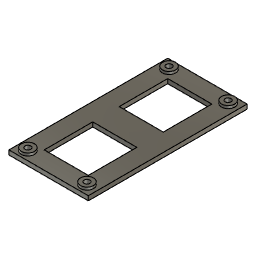
Z axis wheel frame v2 (Autodesk Fusion 360 design; units mm, degrees)
Autodesk Fusion 360 part; units mm, degrees
sketch "Sketch1" plane through (0, 0, 0) normal (0, 1, 0) x (1, 0, 0)
  line L0 (0, -180) -> (0, 0) construction
  line L1 (0, -90) -> (0, -170) construction
  line L2 (0, -170) -> (33.5, -170) construction
  line L3 (45, 0) -> (-45, 0)
  line L4 (-45, 0) -> (-45, -180)
  line L5 (-45, -180) -> (45, -180)
  line L6 (45, -180) -> (45, 0)
  line L7 (0, -170) -> (-33.5, -170) construction
  line L8 (0, -90) -> (0, -10) construction
  line L9 (0, -10) -> (33.5, -10) construction
  line L10 (0, -10) -> (-33.5, -10) construction
  line L11 (-25, -160) -> (25, -160)
  line L12 (25, -160) -> (25, -20)
  line L13 (25, -20) -> (-25, -20)
  line L14 (-25, -20) -> (-25, -160)
  line L15 (-25, -100) -> (25, -100)
  line L16 (25, -75) -> (-25, -75)
  circle A0 centre (33.5, -170) radius 7.5
  circle A1 centre (-33.5, -170) radius 7.5
  circle A2 centre (33.5, -10) radius 7.5
  circle A3 centre (-33.5, -10) radius 7.5
  dimension "d6" = 80
  dimension "d7" = 33.5
  dimension "d8" = 90
  dimension "d9" = 180
  dimension "d10" = 33.5
  dimension "d11" = 80
  dimension "d12" = 33.5
  dimension "d13" = 33.5
  dimension "d14" = 15
  dimension "d15" = 15
  dimension "d16" = 15
  dimension "d17" = 15
  constraint coincident L0.end origin
  constraint midpoint L0 L1.start
  constraint perpendicular L0 L2
  constraint horizontal L3
  constraint vertical L4
  constraint horizontal L5
  constraint vertical L6
  constraint perpendicular L1 L7
  constraint parallel L0 L8
  constraint perpendicular L8 L9
  constraint perpendicular L0 L10
  constraint horizontal L11
  constraint vertical L12
  constraint horizontal L13
  constraint vertical L14
  constraint coincident L14 L15.start
  constraint coincident L12 L15.end
  constraint perpendicular L12 L15
  constraint coincident L12 L16.start
  constraint coincident L14 L16.end
  constraint perpendicular L14 L16
  constraint coincident L2.end A0.centre
  constraint coincident L7.end A1.centre
  constraint coincident L9.end A2.centre
  constraint coincident L10.end A3.centre
  measures "d6" distance of L1.start L1.end
  measures "d7" distance of L1.end L2.end
  measures "d8" distance of L3.start L3.end
  measures "d9" distance of L3.start L5.end
  measures "d10" distance of L1.end L7.end
  measures "d11" distance of L1.start L8.end
  measures "d12" distance of L8.end L9.end
  measures "d13" distance of L8.end L10.end
  measures "d14" diameter of A0
  measures "d15" diameter of A1
  measures "d16" diameter of A2
  measures "d17" diameter of A3
extrude "Extrude1" add sketch "Sketch1" against normal blind 5
extrude "Extrude2" add sketch "Sketch1" against normal blind 8 contours A0 | A1 | A2 | A3
hole "Hole1" at (-33.5, 0, 10) at (33.5, 0, 10) at (33.5, 0, 170) at (-33.5, 0, 170) direction (0, -1, 0) diameter 6.6 depth 8 tip angle 180
extrude "Extrude3" add sketch "Sketch1" against normal blind 5 contours L12 L14 L15 L16
move_body "Align1" bodies 1 to x (1, 0, 0) y (0, 0, -1) z (0, 1, 0) at (0, -90, 0)
extrude "Extrude4" add 1 faces at (-8.3333, 10, 1.6667) along direction (0, 1, 0) blind 5
